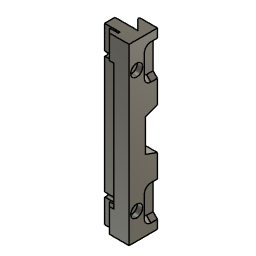
plate attacment v3 v2 (Autodesk Fusion 360 design; units mm, degrees)
Autodesk Fusion 360 part; units mm, degrees
sketch "Sketch1" plane through (0, 0, 0) normal (0, 0, 1) x (1, 0, 0)
  line L0 (4, 0) -> (15, 0)
  line L1 (15, 0) -> (15, 13)
  line L2 (0, 7.5) -> (0, 2)
  line L3 (15, 13) -> (15, 7.5) construction
  line L4 (15, 7.5) -> (0, 7.5) construction
  line L5 (0, 7.5) -> (0, 2.75) construction
  line L6 (0, 2.75) -> (8, 2.75)
  line L7 (8, 2.75) -> (8, 2)
  line L8 (8, 2) -> (0, 2)
  line L9 (0, 2) -> (0, 2.75)
  line L10 (0, 7.5) -> (11.5, 7.5)
  line L11 (4, 2) -> (4, 0)
  line L12 (11.5, 7.5) -> (6, 13)
  line L13 (11.5, 7.5) -> (19.2782, 7.5) construction
  line L14 (6, 13) -> (15, 13)
  dimension "d1" = 15
  dimension "d6" = 8
  dimension "d7" = 0.75
  dimension "d65" = 2
  dimension "d85" = 45
  constraint horizontal L0
  constraint vertical L1
  constraint vertical L2
  constraint vertical L3
  constraint horizontal L4
  constraint perpendicular L4 L5
  constraint horizontal L6
  constraint vertical L7
  constraint horizontal L8
  constraint vertical L9
  constraint coincident L4 L10.end
  constraint midpoint L8 L11.start
  constraint perpendicular L0 L11
  constraint horizontal L13
  measures "d1" distance of origin L0.end
  measures "d6" distance of L5.end L6.end
  measures "d7" distance of L5.end L2.end
  measures "d65" distance of L0 L8
  measures "d85" angle of L12 L13
extrude "Extrude1" add sketch "Sketch1" along normal blind 80
sketch "Sketch2" plane through (15, 0, 0) normal (1, 0, 0) x (0, 1, 0)
  line L0 (0, 0) -> (13, 0)
  line L1 (13, 80) -> (0, 80)
  line L2 (0, 40) -> (15.5, 40) construction
  line L3 (7.5, 47.5) -> (15.5, 47.5)
  line L4 (15.5, 47.5) -> (15.5, 32.5)
  line L5 (15.5, 32.5) -> (7.5, 32.5)
  line L6 (7.5, 32.5) -> (7.5, 47.5)
  line L7 (7.5, 40) -> (15.5, 40) construction
  line L8 (0, 80) -> (0, 0)
  line L9 (13, 0) -> (13, 80)
  dimension "d10" = 8
  dimension "d11" = 15
  constraint horizontal L3
  constraint vertical L4
  constraint horizontal L5
  constraint vertical L6
  constraint midpoint L6 L7.start
  constraint midpoint L4 L2.end
  constraint collinear L2 L7
  measures "d10" distance of L3.start L3.end
  measures "d11" distance of L3.start L5.end
sketch "Sketch4" plane through (15, 0, 0) normal (1, 0, 0) x (0, 1, 0)
  line L0 (13, 80) -> (0, 80)
  line L1 (0, 0) -> (13, 0)
  circle A0 centre (3.5, 68) radius 1.25
  circle A1 centre (3.5, 68) radius 2.75
  line L2 (0, 80) -> (0, 0)
  line L3 (0, 40) -> (15.5, 40) construction
  circle A2 centre (3.5, 12) radius 2.75
  circle A3 centre (3.5, 12) radius 1.25
  line L4 (13, 0) -> (13, 80)
  line L5 (13, 76) -> (10, 76)
  line L6 (7, 73) -> (7, 63)
  line L7 (10, 60) -> (13, 60)
  line L8 (13, 60) -> (13, 76)
  line L9 (7, 68) -> (13, 68) construction
  arc A4 (10, 76) -> (7, 73) centre (10, 73) ccw
  arc A5 (7, 63) -> (10, 60) centre (10, 63) ccw
  line L10 (7, 7) -> (7, 17)
  arc A6 (10, 20) -> (7, 17) centre (10, 17) ccw
  line L11 (10, 20) -> (13, 20)
  line L12 (13, 20) -> (13, 4)
  arc A7 (7, 7) -> (10, 4) centre (10, 7) ccw
  line L13 (13, 4) -> (10, 4)
  dimension "d33" = 2.5
  dimension "d37" = 5.5
  dimension "d40" = 12
  dimension "d81" = 3.5
  dimension "d95" = 16
  dimension "d96" = 3
  constraint concentric A0 A1
  constraint midpoint L2 L3.start
  constraint symmetric A0 L3 A3
  constraint symmetric A1 L3 A2
  constraint horizontal L5
  constraint vertical L6
  constraint horizontal L7
  constraint vertical L8
  constraint coincident L4 L5.start
  constraint midpoint L8 L9.end
  constraint coincident A0.centre L9
  constraint coincident L6 L9.start
  constraint tangent L5 A4
  constraint tangent L6 A4
  constraint tangent L7 A5
  constraint tangent L6 A5
  constraint equal A4 A5
  constraint symmetric L3 L5.start L12.end
  constraint symmetric L3 L7.end L11.end
  constraint symmetric L3 L5.end A7.end
  constraint symmetric L3 L6.start L10.start
  constraint symmetric L3 A4 A7
  constraint symmetric L3 L7.start A6.start
  constraint symmetric L3 L6.end L10.end
  constraint symmetric L3 A5 A6
  measures "d33" diameter of A0
  measures "d37" diameter of A1
  measures "d40" distance of L0 A0.centre
  measures "d81" distance of A0.centre L2
  measures "d95" distance of L5.start L7.end
  measures "d96" radius of A4
sketch "Sketch5" plane through (0, 0, 0) normal (0, -1, 0) x (1, 0, 0)
  line L0 (4, 0) -> (15, 0)
  line L1 (15, 0) -> (15, 80)
  line L2 (15, 80) -> (4, 80)
  circle A0 centre (4.5, 71.5) radius 1.25
  line L3 (15, 40) -> (0, 40) construction
  line L4 (0, 69) -> (8, 69)
  line L5 (8, 69) -> (8, 11)
  line L6 (8, 11) -> (0, 11)
  line L7 (0, 11) -> (0, 69)
  line L8 (0, 40) -> (8, 40) construction
  line L9 (4, 80) -> (4, 0)
  dimension "d45" = 2.5
  dimension "d46" = 8.5
  dimension "d51" = 8
  dimension "d52" = 58
  constraint midpoint L1 L3.start
  constraint horizontal L4
  constraint vertical L5
  constraint horizontal L6
  constraint vertical L7
  constraint midpoint L7 L3.end
  constraint midpoint L5 L8.end
  constraint collinear L3 L8
  measures "d45" diameter of A0
  measures "d46" distance of L2 A0.centre
  measures "d51" distance of L4.start L4.end
  measures "d52" distance of L4.start L6.end
extrude "Extrude9" cut sketch "Sketch5" against normal blind 11 contours A0 L9 | A0 L9
extrude "Extrude10" cut sketch "Sketch5" against normal blind 2.5 contours L4 L5 L6 L9 | L4 L6 L7 L9
extrude "Extrude14" cut 1 faces at (0, 5.8333, 49.6667) along direction (1, 0, 0) blind 1
chamfer "Chamfer5" distance 2 angle 45 3 edges at (4, 0, 69.6772) (4, 0, 76.3228) (4, 0, 5.5)
extrude "Extrude15" cut sketch "Sketch2" against normal blind 10 contours L3 L4 L5 L9 | L3 L5 L6 L9
extrude "Extrude17" cut sketch "Sketch4" against normal blind 14 contours A0 | A3
extrude "Extrude18" add sketch "Sketch4" against normal blind 2.75 contours A0 | A3
extrude "Extrude19" cut sketch "Sketch4" against normal blind 2.5 contours A0 | A1 | A2 | A3
extrude "Extrude20" cut sketch "Sketch1" along normal blind 80 contours L2 L6 L7 L8 L9
chamfer "Chamfer8" distance 2 distance2 5.5 2 edges at (10.5, 13, 47.5) (10.5, 13, 32.5) measured on face at (12, 13, 69.1667) measured on face at (12, 13, 10.8333)
fillet "Fillet5" radius 0.5 2 edges at (6, 13, 64.75) (6, 13, 15.25)
extrude "Extrude21" cut sketch "Sketch4" against normal blind 2 contours L4 L5 L6 L7 L8 A4 A5 | L4 L10 A6 L11 L12 A7 L13
chamfer "Chamfer10" distance 2 angle 45 10 edges at (13, 7.8787, 19.1213) (13, 11.5, 20) (13, 11.5, 4) (13, 7.8787, 4.8787) (13, 7, 12) (13, 7, 68) (13, 7.8787, 75.1213) (13, 11.5, 76) (13, 11.5, 60) (13, 7.8787, 60.8787)
